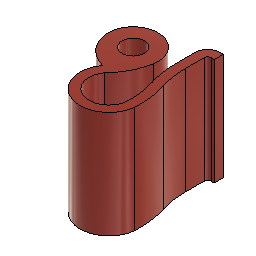
Day3 - Filament clip reverse engineered (Autodesk Fusion 360 design; units mm, degrees)
Autodesk Fusion 360 part; units mm, degrees
mesh "Mesh1" [no effect]
sketch "Sketch1" plane through (0, 0, 0.5) normal (0, 0, 1) x (1, 0, 0)
  line L0 (10, 6.849) -> (9.9833, 5.409)
  line L1 (9.9833, 5.409) -> (9.5, 5.409)
  arc A0 (9.5, 5.409) -> (8.9402, 4.8522) centre (9.5002, 4.8489) ccw
  line L2 (8.9402, 4.8522) -> (8.94, 1.849)
  arc A1 (8.94, 1.849) -> (9.553, -2.1826) centre (22.5715, 1.8593) ccw
  arc A2 (9.553, -2.1826) -> (10.2442, -7.4574) centre (-5.1993, -6.7983) cw
  arc A3 (10.2442, -7.4574) -> (1.9534, -4.2546) centre (5.6628, -6.9847) cw
  line L3 (9.5, 6.849) -> (10, 6.849)
  arc A4 (7.5004, 4.849) -> (9.5, 6.849) centre (9.5009, 4.8485) cw
  line L4 (7.5, 1.849) -> (7.5004, 4.849)
  arc A5 (8.1759, -2.6032) -> (7.5, 1.849) centre (22.5735, 1.8599) cw
  arc A6 (8.798, -7.4258) -> (8.1759, -2.6032) centre (-4.8987, -6.7413) ccw
  arc A7 (3.086, -5.1438) -> (8.798, -7.4258) centre (5.6627, -6.9839) ccw
  arc A8 (3.086, -5.1438) -> (5.7392, 0.0083) centre (-3.8214, 1.6727) ccw
  arc A9 (5.7392, 0.0083) -> (-2.0626, 0.0086) centre (1.8383, 0.6874) ccw
  arc A10 (-2.0626, 0.0086) -> (1.9534, -4.2546) centre (3.1758, 0.9201) ccw
  circle A11 centre (1.8383, 0.6874) radius 1.75
  dimension "d1" = 3.5
  measures "d1" diameter of A11
extrude "Extrude1" add sketch "Sketch1" along normal blind 17
named bodies: "filament clip"
